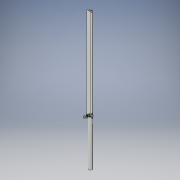
# Autodesk Inventor part: L60x2profilSas
Saved by Autodesk Inventor 2019 (Build 230136000, 136)
## iProperties
Created: 2025-01-08
Part Number: L60x2profilSas
Material: Generic
Document SubType Name: Modeling
Designer: laca
Density: 1 g/cm^3
Appearance: Default
Mass: 4730.81 g
Surface Area: 18525.9 cm^2
Volume: 4730.81 cm^3
Author: laca
Autodesk Inventor part; units mm, degrees
ref_plane "YZ Plane" through (0, 0, 0) normal (1, 0, 0) x (0, 1, 0)
ref_plane "XZ Plane" through (0, 0, 0) normal (0, 1, 0) x (-1, 0, 0)
ref_plane "XY Plane" through (0, 0, 0) normal (0, 0, 1) x (1, 0, 0)
sketch "Sketch1" plane through (0, 0, 0) normal (0, 1, 0) x (-1, 0, 0)
  line L0 (0, 0) -> (0, 60)
  line L1 (0, 60) -> (60, 60)
  line L2 (56, 55) -> (9, 55)
  line L3 (5, 51) -> (5, 4)
  line L4 (60, 60) -> (60, 59)
  line L5 (0, 0) -> (1, 0)
  arc A0 (1, 0) -> (5, 4) centre (1, 4) ccw
  arc A1 (56, 55) -> (60, 59) centre (56, 59) ccw
  arc A2 (9, 55) -> (5, 51) centre (9, 51) ccw
  line L6 (5, 30) -> (35, 30)
  line L7 (35, 30) -> (35, 26)
  line L8 (35, 26) -> (5, 26)
  line L9 (0, 60) -> (-60, 60)
  line L10 (-56, 55) -> (-9, 55)
  line L11 (-5, 51) -> (-5, 4)
  line L12 (-60, 60) -> (-60, 59)
  line L13 (0, 0) -> (-1, 0)
  arc A3 (-5, 4) -> (-1, 0) centre (-1, 4) ccw
  arc A4 (-60, 59) -> (-56, 55) centre (-56, 59) ccw
  arc A5 (-5, 51) -> (-9, 55) centre (-9, 51) ccw
  line L14 (-5, 30) -> (-35, 30)
  line L15 (-35, 30) -> (-35, 26)
  line L16 (-35, 26) -> (-5, 26)
  circle A6 centre (0, 41.935) radius 40
  circle A7 centre (0, 41.935) radius 37
  dimension "d0" = 60
  dimension "d1" = 60
  dimension "d2" = 5
  dimension "d3" = 4
  dimension "d4" = 30
  dimension "d5" = 4
  dimension "d6" = 25
  dimension "d9" = 80
  dimension "d10" = 3
  constraints: 34 end point, 14 symmetric about line, 12 point on circle, 8 centre point, 6 tangent, 5 point on line, 3 perpendicular, 2 equal radius, 2 horizontal, 2 vertical, 4 other
  measures "d0" distance of L0.start L0.end
  measures "d1" distance of L0.end L1.end
  measures "d2" distance between parallel lines of L1 L2
  measures "d3" radius of A0
  measures "d4" distance of L6.start L6.end
  measures "d5" distance of L6.end L7.end
  measures "d6" distance between parallel lines of L2 L6
  measures "d9" diameter of A6
  measures "d10" radial gap between concentric circles of A7 A6
extrude "Extrusion1" add sketch "Sketch1" along normal blind 2000 contours L13 A3 A6 L0 | L0 A6 A0 L5 | A6 A3 L11 A7 L0 | L0 A7 L3 A0 A6 | A7 L11 A5 L10 L9 L0 | L0 L1 A7 L2 A2 L3 | A6 L9 A7 L10 | L10 A4 L12 L9 A6 | L1 A6 L2 A7 | L16 A7 L15 L14 L11 | L16 L15 A7 | L3 L6 L7 A7 L8 | A7 L7 L8 | A6 L1 L4 A1 L2
extrude "Extrusion2" add sketch "Sketch1" against normal blind 1000 contours A6 A3 L11 A7 L0 | L0 A7 L3 A0 A6 | A6 L10 A7 L15 L16 L11 A3 | A0 L3 A7 L8 L7 L2 A6 | A6 L9 A7 L10 | A7 L9 A6 L1 | L1 A6 L2 A7
body "Solid1"
